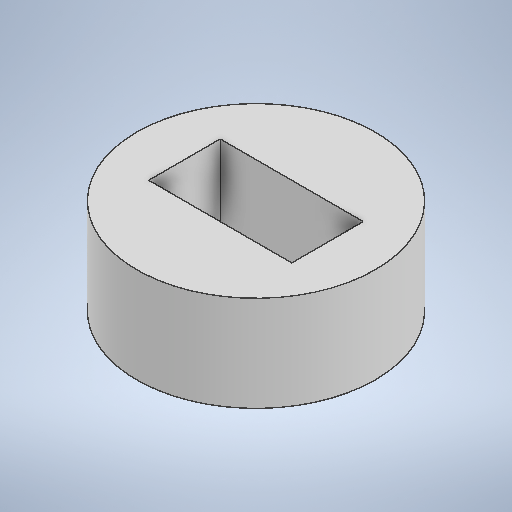
# Autodesk Inventor part: plate_ball
Saved by Autodesk Inventor 2025 (Build 290162000, 162)
## iProperties
Created: 2025-10-18
Part Number: plate_ball
Material: 一般
Document SubType Name: Modeling
Designer: sooo1
Density: 1 g/cm^3
Appearance: 既定
Author: sooo1
Autodesk Inventor part; units mm, degrees
ref_plane "YZ Plane" through (0, 0, 0) normal (1, 0, 0) x (0, 1, 0)
ref_plane "XZ Plane" through (0, 0, 0) normal (0, 1, 0) x (-1, 0, 0)
ref_plane "XY Plane" through (0, 0, 0) normal (0, 0, 1) x (1, 0, 0)
sketch "スケッチ1" plane through (0, 0, 0) normal (0, 1, 0) x (-1, 0, 0)
  circle A0 centre (0, 0) radius 2.5
  line L0 (1.5, 0.75) -> (-1.5, 0.75)
  line L1 (-1.5, 0.75) -> (-1.5, -0.75)
  line L2 (-1.5, -0.75) -> (1.5, -0.75)
  line L3 (1.5, -0.75) -> (1.5, 0.75)
  line L4 (1.5, 0.75) -> (-1.5, -0.75) construction
  line L5 (-1.5, 0.75) -> (1.5, -0.75) construction
  dimension "d0" = 5
  dimension "d1" = 1.5
  dimension "d2" = 3
  constraints: 12 end point, 2 midpoint, 2 parallel, 1 centre point, 1 coincident, 1 horizontal, 1 perpendicular
  measures "d0" diameter of A0
  measures "d1" distance of L2.end L0.start
  measures "d2" distance of L1.end L2.end
extrude "押し出し1" add sketch "スケッチ1" along normal blind 2
